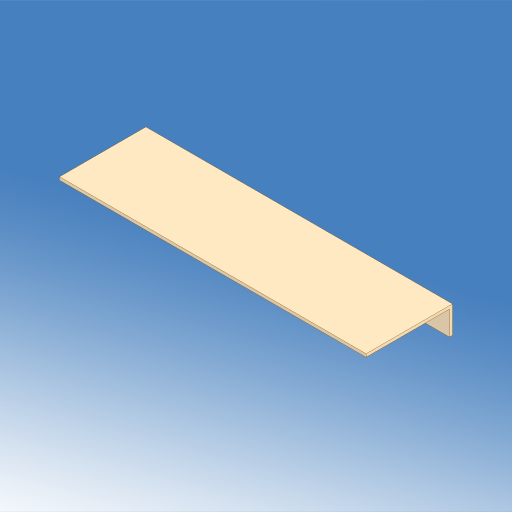
# Autodesk Inventor part: flat chain guide
Saved by Autodesk Inventor 2024 (Build 280153000, 153)
## iProperties
Created: 2023-03-01
Part Number: flat chain guide
Material: Polyethylene, High Density
Document SubType Name: Modeling
Designer: ralph
Density: 0.952 g/cm^3
Appearance: Smooth - Off-White
Author: ralph
Autodesk Inventor part; units mm, degrees
ref_plane "Work Plane1" through (-105.5469, -33.8995, 0) normal (0, 0, 1) x (1, 0, 0)
sketch "Sketch1" plane through (-105.5469, -33.8995, 0) normal (0, 0, 1) x (1, 0, 0)
  circle A0 centre (51.4164, 20.6909) radius 2.413 projected
  circle A1 centre (61.5426, -29.0897) radius 2.413 projected
  circle A2 centre (41.2902, 70.4714) radius 2.413 projected
  circle A3 centre (71.6688, -78.8702) radius 2.413 projected
  circle A4 centre (27.8827, -36.0288) radius 3.175 projected
  line L0 (21.5564, -145.7309) -> (-91.4082, 76.2381) projected
  line L1 (59.5069, 74.2446) -> (98.755, -118.7966) projected
  line L2 (15.2228, 144.056) -> (44.9436, 105.9012) projected
  line L3 (63.6348, -131.723) -> (58.903, -119.9375) projected
  line L4 (53.0129, -122.3028) -> (57.7447, -134.0883) projected
  arc A5 (3.7348, 135.3868) -> (-79.7406, 82.2913) centre (-35.4587, 104.8391) ccw
  line L5 (3.7348, 135.3868) -> (33.4679, 97.2384)
  arc A6 (45.3974, 71.3204) -> (33.4679, 97.2384) centre (-15.7425, 58.8835) ccw
  line L6 (45.3974, 71.3204) -> (84.6647, -121.7179)
  arc A7 (33.2723, -139.6562) -> (84.6647, -121.7179) centre (57.7489, -127.193) ccw
  arc A8 (2.9524, 134.777) -> (-78.8566, 82.7414) centre (-35.4587, 104.8391) ccw
  line L7 (2.9524, 134.777) -> (32.6855, 96.6286)
  arc A9 (44.4253, 71.1227) -> (32.6855, 96.6286) centre (-15.7425, 58.8835) ccw
  line L8 (44.4253, 71.1227) -> (83.6926, -121.9156)
  arc A10 (34.1563, -139.2061) -> (83.6926, -121.9156) centre (57.7489, -127.193) ccw
  line L9 (34.1563, -139.2061) -> (-78.8566, 82.7414)
  arc A11 (-4.5602, 128.9216) -> (-70.3686, 87.0634) centre (-35.4587, 104.8391) ccw
  line L10 (-4.5602, 128.9216) -> (25.1729, 90.7732)
  arc A12 (35.0915, 69.224) -> (25.1729, 90.7732) centre (-15.7425, 58.8835) ccw
  line L11 (35.0915, 69.224) -> (74.3588, -123.8143)
  arc A13 (42.6443, -134.8841) -> (74.3588, -123.8143) centre (57.7489, -127.193) ccw
  line L12 (42.6443, -134.8841) -> (-70.3686, 87.0634)
  arc A14 (5.4566, 136.7288) -> (-81.686, 81.3007) centre (-35.4587, 104.8391) ccw
  line L13 (5.4566, 136.7288) -> (35.1897, 98.5804)
  arc A15 (47.5366, 71.7556) -> (35.1897, 98.5804) centre (-15.7425, 58.8835) ccw
  line L14 (47.5366, 71.7556) -> (86.8039, -121.2827)
  arc A16 (31.327, -140.6467) -> (86.8039, -121.2827) centre (57.7489, -127.193) ccw
  line L15 (31.327, -140.6467) -> (-81.686, 81.3007)
  circle A17 centre (57.7489, -127.193) radius 44.45
  circle A18 centre (-35.4587, 104.8391) radius 69.85
  circle A19 centre (-47.8242, 28.7936) radius 2.413 projected
  circle A20 centre (-15.5534, -34.5834) radius 2.413 projected
  circle A21 centre (16.7174, -97.9605) radius 2.413 projected
  line L16 (-33.1344, 24.0942) -> (34.7456, 18.5458) projected
  line L17 (36.5081, 12.9323) -> (-6.2049, -22.3208) projected
  line L18 (-20.7511, -20.2117) -> (-39.1333, 15.9083) projected
  line L19 (38.3036, 25.8999) -> (-20.4951, 30.706) projected
  line L20 (-21.5821, 36.7465) -> (30.7819, 61.2351) projected
  line L21 (44.0707, 55.5202) -> (48.097, 35.7165) projected
  line L22 (-53.0081, 43.1715) -> (-61.3301, 59.5239) projected
  line L23 (17.8998, 109.9146) -> (30.1007, 94.2514) projected
  line L24 (27.5547, 68.1378) -> (-5.8444, 52.5185) projected
  line L25 (27.1825, -114.3985) -> (25.3807, -110.8581) projected
  line L26 (32.1964, -96.6363) -> (38.137, -94.5724) projected
  line L27 (74.4344, -93.8236) -> (75.2107, -97.6416) projected
  line L28 (50.495, -96.7953) -> (49.4394, -94.1661) projected
  line L29 (51.3425, -89.9843) -> (60.23, -86.8964) projected
  line L30 (-10.1341, 54.212) -> (-12.6231, 60.4113) projected
  line L31 (-19.6913, 57.573) -> (-16.9128, 50.6526) projected
  line L32 (-18.5132, 46.5938) -> (-35.734, 38.5403) projected
  line L33 (42.124, -96.3889) -> (43.4268, -99.6336) projected
  arc A22 (40.3328, 7.2327) -> (41.7343, 8.6241) centre (33.4597, 15.5569) ccw projected
  arc A23 (45.6191, 9.409) -> (41.7343, 8.6241) centre (44.1679, 6.585) ccw projected
  arc A24 (45.6191, 9.409) -> (50.3997, 8.0475) centre (51.4164, 20.6909) ccw projected
  arc A25 (53.2564, 5.5162) -> (50.3997, 8.0475) centre (50.1452, 4.8827) ccw projected
  line L34 (53.2564, 5.5162) -> (57.2026, -13.8642) projected
  arc A26 (55.534, -17.3261) -> (57.2026, -13.8642) centre (54.0915, -14.4977) ccw projected
  arc A27 (55.534, -17.3261) -> (49.5198, -23.895) centre (61.311, -28.6529) ccw projected
  arc A28 (46.8024, -25.8738) -> (49.5198, -23.895) centre (46.5755, -22.7069) ccw projected
  line L35 (46.8024, -25.8738) -> (37.6772, -26.5277) projected
  arc A29 (35.5367, -25.8944) -> (37.6772, -26.5277) centre (37.4502, -23.3608) ccw projected
  arc A30 (35.5367, -25.8944) -> (18.8618, -27.0893) centre (27.8827, -36.0288) ccw projected
  arc A31 (16.8336, -28.0213) -> (18.8618, -27.0893) centre (16.6066, -24.8545) ccw projected
  line L36 (16.8336, -28.0213) -> (0.7655, -29.1728) projected
  arc A32 (-0.3587, -26.3652) -> (0.7655, -29.1728) centre (0.652, -27.5893) ccw projected
  line L37 (-0.3587, -26.3652) -> (40.3328, 7.2327) projected
  arc A33 (12.0706, -61.7398) -> (8.1483, -51.9706) centre (20.8352, -52.5488) ccw projected
  line L38 (25.9855, -70.6908) -> (17.4507, -83.8024) projected
  line L39 (11.5059, -83.5949) -> (-6.8763, -47.4749) projected
  line L40 (-0.2859, -37.1185) -> (-0.1921, -37.1119) projected
  line L41 (74.8789, -123.628) -> (78.6564, -122.8604) projected
  line L42 (0.38, 132.4063) -> (2.0588, 130.251) projected
  line L43 (38.7029, -137.0353) -> (37.8849, -135.428) projected
  line L44 (38.579, -133.2932) -> (44.3373, -130.3617) projected
  line L45 (12.0706, -61.7398) -> (13.7631, -65.9552) projected
  line L46 (17.8911, -67.7189) -> (22.1428, -66.0115) projected
  line L47 (2.9792, -39.0961) -> (8.1483, -51.9706) projected
  ellipse E0 centre (-34.8429, 105.035) end of major axis (-54.1736, 165.5211) minor radius 63.4728 (15.2228, 144.056) -> (-91.4082, 76.2381) ccw projected
  ellipse E1 centre (58.3238, -127.0129) end of major axis (45.7589, -87.6969) minor radius 41.2573 (21.5564, -145.7309) -> (98.755, -118.7966) ccw projected
  ellipse E2 centre (-15.1352, 59.076) end of major axis (-38.3321, 131.6593) minor radius 76.1674 (59.5069, 74.2446) -> (44.9436, 105.9012) ccw projected
  ellipse E3 centre (-34.8429, 105.035) end of major axis (-38.9507, 117.8883) minor radius 13.488 projected
  ellipse E4 centre (60.6898, -132.9057) end of major axis (59.7232, -129.8814) minor radius 3.1736 (57.7447, -134.0883) -> (63.6348, -131.723) ccw projected
  ellipse E5 centre (55.9579, -121.1202) end of major axis (54.9914, -118.0958) minor radius 3.1736 (58.903, -119.9375) -> (53.0129, -122.3028) ccw projected
  ellipse E6 centre (-47.0283, 29.0524) end of major axis (-50.8944, 41.1496) minor radius 12.6946 (-38.4497, 19.689) -> (-36.1193, 22.5544) ccw projected
  ellipse E7 centre (-33.3921, 20.9299) end of major axis (-34.3586, 23.9542) minor radius 3.1736 (-33.1344, 24.0942) -> (-36.1193, 22.5544) ccw projected
  ellipse E8 centre (34.4879, 15.3814) end of major axis (33.5214, 18.4057) minor radius 3.1736 (36.5081, 12.9323) -> (34.7456, 18.5458) ccw projected
  ellipse E9 centre (-8.2251, -19.8717) end of major axis (-7.2586, -22.896) minor radius 3.1736 (-9.5343, -22.7635) -> (-6.2049, -22.3208) ccw projected
  ellipse E10 centre (-14.7713, -34.3308) end of major axis (-18.6374, -22.2336) minor radius 12.6946 (-9.5343, -22.7635) -> (-17.2925, -21.8836) ccw projected
  ellipse E11 centre (-17.9228, -18.7718) end of major axis (-16.9563, -21.7962) minor radius 3.1736 (-20.7511, -20.2117) -> (-17.2925, -21.8836) ccw projected
  ellipse E12 centre (-36.305, 17.3481) end of major axis (-35.3385, 14.3238) minor radius 3.1736 (-38.4497, 19.689) -> (-39.1333, 15.9083) ccw projected
  ellipse E13 centre (38.5613, 29.0642) end of major axis (39.5278, 26.0399) minor radius 3.1736 (38.3036, 25.8999) -> (41.2885, 27.4397) ccw projected
  ellipse E14 centre (-20.2374, 33.8704) end of major axis (-19.2708, 30.8461) minor radius 3.1736 (-21.5821, 36.7465) -> (-20.4951, 30.706) ccw projected
  ellipse E15 centre (32.1266, 58.3589) end of major axis (31.1601, 61.3832) minor radius 3.1736 (34.1165, 60.8317) -> (30.7819, 61.2351) ccw projected
  ellipse E16 centre (42.0762, 70.723) end of major axis (38.2101, 82.8202) minor radius 12.6946 (34.1165, 60.8317) -> (41.1837, 58.0551) ccw projected
  ellipse E17 centre (40.9606, 54.8882) end of major axis (39.994, 57.9125) minor radius 3.1736 (44.0707, 55.5202) -> (41.1837, 58.0551) ccw projected
  ellipse E18 centre (44.9869, 35.0845) end of major axis (44.0204, 38.1088) minor radius 3.1736 (46.4291, 32.2559) -> (48.097, 35.7165) ccw projected
  ellipse E19 centre (-37.0786, 41.4165) end of major axis (-36.1121, 38.3922) minor radius 3.1736 (-39.0686, 38.9437) -> (-35.734, 38.5403) ccw projected
  ellipse E20 centre (-47.0283, 29.0524) end of major axis (-50.8944, 41.1496) minor radius 12.6946 (-39.0686, 38.9437) -> (-49.5495, 41.4996) ccw projected
  ellipse E21 centre (-50.1798, 44.6113) end of major axis (-49.2133, 41.587) minor radius 3.1736 (-53.0081, 43.1715) -> (-49.5495, 41.4996) ccw projected
  ellipse E22 centre (-58.5019, 60.9637) end of major axis (-57.5353, 57.9394) minor radius 3.1736 (-56.9933, 63.7566) -> (-61.3301, 59.5239) ccw projected
  ellipse E23 centre (-34.666, 105.0915) end of major axis (-48.9707, 149.8513) minor radius 46.9699 (-11.2596, 64.347) -> (12.228, 107.7818) ccw projected
  ellipse E24 centre (15.3966, 107.9636) end of major axis (14.43, 110.9879) minor radius 3.1736 (17.8998, 109.9146) -> (12.228, 107.7818) ccw projected
  ellipse E25 centre (-14.9584, 59.1325) end of major axis (2.4393, 4.6949) minor radius 57.1256 (35.8618, 85.223) -> (30.1007, 94.2514) ccw projected
  ellipse E26 centre (33.0385, 83.7735) end of major axis (32.0719, 86.7978) minor radius 3.1736 (34.846, 81.1634) -> (35.8618, 85.223) ccw projected
  ellipse E27 centre (42.0762, 70.723) end of major axis (38.2101, 82.8202) minor radius 12.6946 (34.846, 81.1634) -> (29.3832, 70.9558) ccw projected
  ellipse E28 centre (26.21, 71.014) end of major axis (25.2435, 74.0383) minor radius 3.1736 (27.5547, 68.1378) -> (29.3832, 70.9558) ccw projected
  ellipse E29 centre (58.5007, -126.9564) end of major axis (49.8019, -99.7376) minor radius 28.5628 (70.7406, -101.1419) -> (53.9461, -98.747) ccw projected
  ellipse E30 centre (30.0108, -112.9586) end of major axis (30.9773, -115.9829) minor radius 3.1736 (27.1825, -114.3985) -> (32.8598, -114.3584) ccw projected
  ellipse E31 centre (28.209, -109.4182) end of major axis (29.1755, -112.4425) minor radius 3.1736 (26.0643, -107.0774) -> (25.3807, -110.8581) ccw projected
  ellipse E32 centre (17.4857, -97.714) end of major axis (21.3519, -109.8112) minor radius 12.6946 (26.0643, -107.0774) -> (30.0878, -99.2512) ccw projected
  ellipse E33 centre (33.2384, -99.6355) end of major axis (34.2049, -102.6598) minor radius 3.1736 (32.1964, -96.6363) -> (30.0878, -99.2512) ccw projected
  ellipse E34 centre (61.272, -89.8956) end of major axis (60.3054, -86.8713) minor radius 3.1736 (63.5056, -87.6406) -> (60.23, -86.8964) ccw projected
  ellipse E35 centre (72.44, -78.6208) end of major axis (68.5739, -66.5236) minor radius 12.6946 (63.5056, -87.6406) -> (71.5475, -91.2887) ccw projected
  ellipse E36 centre (71.3244, -94.4556) end of major axis (70.3578, -91.4313) minor radius 3.1736 (74.4344, -93.8236) -> (71.5475, -91.2887) ccw projected
  ellipse E37 centre (72.1006, -98.2736) end of major axis (73.0671, -101.2979) minor radius 3.1736 (70.7406, -101.1419) -> (75.2107, -97.6416) ccw projected
  ellipse E38 centre (58.5007, -126.9564) end of major axis (49.8019, -99.7376) minor radius 28.5628 (42.2836, -103.4303) -> (32.8598, -114.3584) ccw projected
  ellipse E39 centre (-34.666, 105.0915) end of major axis (-48.9707, 149.8513) minor radius 46.9699 (-56.9933, 63.7566) -> (-23.3977, 59.4727) ccw projected
  ellipse E40 centre (53.44, -95.6126) end of major axis (54.4066, -98.6369) minor radius 3.1736 (50.495, -96.7953) -> (53.9461, -98.747) ccw projected
  ellipse E41 centre (52.3844, -92.9835) end of major axis (53.351, -96.0078) minor radius 3.1736 (51.3425, -89.9843) -> (49.4394, -94.1661) ccw projected
  ellipse E42 centre (-7.1891, 55.3946) end of major axis (-6.2225, 52.3703) minor radius 3.1736 (-10.1341, 54.212) -> (-5.8444, 52.5185) ccw projected
  ellipse E43 centre (-9.6781, 61.594) end of major axis (-8.7115, 58.5697) minor radius 3.1736 (-11.2596, 64.347) -> (-12.6231, 60.4113) ccw projected
  ellipse E44 centre (-19.8578, 49.4699) end of major axis (-20.8244, 52.4943) minor radius 3.1736 (-18.5132, 46.5938) -> (-16.9128, 50.6526) ccw projected
  ellipse E45 centre (-22.6364, 56.3903) end of major axis (-23.6029, 59.4146) minor radius 3.1736 (-19.6913, 57.573) -> (-23.3977, 59.4727) ccw projected
  ellipse E46 centre (39.179, -97.5715) end of major axis (38.2124, -94.5472) minor radius 3.1736 (42.124, -96.3889) -> (38.137, -94.5724) ccw projected
  ellipse E47 centre (40.4817, -100.8163) end of major axis (39.5152, -97.792) minor radius 3.1736 (42.2836, -103.4303) -> (43.4268, -99.6336) ccw projected
  ellipse E48 centre (14.791, -82.0695) end of major axis (15.7575, -85.0938) minor radius 3.1736 (15.3299, -85.1984) -> (17.4507, -83.8024) ccw projected
  ellipse E49 centre (17.4857, -97.714) end of major axis (13.6196, -85.6168) minor radius 12.6946 (15.3299, -85.1984) -> (14.9645, -85.2668) ccw projected
  ellipse E50 centre (14.3342, -82.155) end of major axis (15.3007, -85.1793) minor radius 3.1736 (11.5059, -83.5949) -> (14.9645, -85.2668) ccw projected
  ellipse E51 centre (-4.048, -46.035) end of major axis (-3.0815, -49.0593) minor radius 3.1736 (-6.1927, -43.6942) -> (-6.8763, -47.4749) ccw projected
  ellipse E52 centre (-14.7713, -34.3308) end of major axis (-10.9051, -46.428) minor radius 12.6946 (-6.1927, -43.6942) -> (-3.002, -39.0945) ccw projected
  ellipse E53 centre (-0.0597, -40.2854) end of major axis (-1.0262, -37.2611) minor radius 3.1736 (-0.2859, -37.1185) -> (-3.002, -39.0945) ccw projected
  ellipse E54 centre (-75.9068, 106.3278) end of major axis (-76.8733, 109.3521) minor radius 3.1736 (-73.3969, 108.2703) -> (-79.0792, 106.4229) ccw projected
  ellipse E55 centre (-58.3372, 119.9252) end of major axis (-64.1365, 138.071) minor radius 19.0419 (-73.3969, 108.2703) -> (-70.1692, 105.0022) ccw projected
  ellipse E56 centre (-72.1411, 102.5151) end of major axis (-73.1077, 105.5394) minor radius 3.1736 (-69.8464, 100.3213) -> (-70.1692, 105.0022) ccw projected
  ellipse E57 centre (-56.078, 87.1583) end of major axis (-61.8772, 105.3042) minor radius 19.0419 (-69.8464, 100.3213) -> (-72.5951, 96.6423) ccw projected
  ellipse E58 centre (-75.348, 98.223) end of major axis (-74.3814, 95.1987) minor radius 3.1736 (-78.4773, 97.6947) -> (-72.5951, 96.6423) ccw projected
  ellipse E59 centre (-34.666, 105.0915) end of major axis (-21.1345, 62.7512) minor radius 44.431 (-79.0792, 106.4229) -> (-78.4773, 97.6947) ccw projected
  ellipse E60 centre (-46.2445, 144.7092) end of major axis (-47.211, 147.7336) minor radius 3.1736 (-43.6215, 142.9211) -> (-47.1351, 147.7568) ccw projected
  ellipse E61 centre (-27.8837, 132.1924) end of major axis (-33.6829, 150.3383) minor radius 19.0419 (-43.6215, 142.9211) -> (-45.7303, 138.8412) ccw projected
  ellipse E62 centre (-48.7048, 139.9494) end of major axis (-47.7382, 136.925) minor radius 3.1736 (-50.0809, 137.0888) -> (-45.7303, 138.8412) ccw projected
  ellipse E63 centre (-58.3372, 119.9252) end of major axis (-64.1365, 138.071) minor radius 19.0419 (-50.0809, 137.0888) -> (-54.4286, 138.5679) ccw projected
  ellipse E64 centre (-53.7771, 141.675) end of major axis (-52.8106, 138.6507) minor radius 3.1736 (-55.2472, 144.4891) -> (-54.4286, 138.5679) ccw projected
  ellipse E65 centre (-34.666, 105.0915) end of major axis (-21.1345, 62.7512) minor radius 44.431 (-47.1351, 147.7568) -> (-55.2472, 144.4891) ccw projected
  ellipse E66 centre (78.9727, -124.4161) end of major axis (78.4894, -122.9039) minor radius 1.5868 (80.5474, -124.2206) -> (78.6564, -122.8604) ccw projected
  ellipse E67 centre (58.5007, -126.9564) end of major axis (51.735, -105.7862) minor radius 22.2155 (79.7691, -133.3844) -> (80.5474, -124.2206) ccw projected
  ellipse E68 centre (76.7308, -132.4661) end of major axis (77.6973, -135.4904) minor radius 3.1736 (73.5579, -132.5427) -> (79.7691, -133.3844) ccw projected
  ellipse E69 centre (60.8666, -132.8492) end of major axis (64.7328, -144.9464) minor radius 12.6946 (73.5579, -132.5427) -> (72.5825, -127.9613) ccw projected
  ellipse E70 centre (75.5115, -126.7394) end of major axis (74.545, -123.7151) minor radius 3.1736 (74.8789, -123.628) -> (72.5825, -127.9613) ccw projected
  ellipse E71 centre (-0.4445, 128.2999) end of major axis (0.522, 125.2756) minor radius 3.1736 (-1.3529, 125.2581) -> (2.0588, 130.251) ccw projected
  ellipse E72 centre (-6.8031, 107.0071) end of major axis (-12.6023, 125.153) minor radius 19.0419 (-1.3529, 125.2581) -> (-6.001, 126.0393) ccw projected
  ellipse E73 centre (-5.8673, 129.2113) end of major axis (-4.9008, 126.187) minor radius 3.1736 (-9.0125, 129.6372) -> (-6.001, 126.0393) ccw projected
  ellipse E74 centre (-27.8837, 132.1924) end of major axis (-33.6829, 150.3383) minor radius 19.0419 (-9.0125, 129.6372) -> (-8.9508, 134.2302) ccw projected
  ellipse E75 centre (-5.7954, 134.5699) end of major axis (-6.7619, 137.5942) minor radius 3.1736 (-3.5745, 136.8374) -> (-8.9508, 134.2302) ccw projected
  ellipse E76 centre (-34.666, 105.0915) end of major axis (-21.1345, 62.7512) minor radius 44.431 (0.38, 132.4063) -> (-3.5745, 136.8374) ccw projected
  ellipse E77 centre (39.299, -134.708) end of major axis (39.7823, -136.2202) minor radius 1.5868 (38.579, -133.2932) -> (37.8849, -135.428) ccw projected
  ellipse E78 centre (45.0573, -131.7765) end of major axis (44.5741, -130.2644) minor radius 1.5868 (46.551, -131.2409) -> (44.3373, -130.3617) ccw projected
  ellipse E79 centre (58.5007, -126.9564) end of major axis (54.6346, -114.8592) minor radius 12.6946 (46.551, -131.2409) -> (48.2775, -134.4832) ccw projected
  ellipse E80 centre (60.8666, -132.8492) end of major axis (64.7328, -144.9464) minor radius 12.6946 (48.2775, -134.4832) -> (51.4877, -141.4055) ccw projected
  ellipse E81 centre (49.1429, -143.5446) end of major axis (48.1764, -140.5202) minor radius 3.1736 (47.5833, -146.3092) -> (51.4877, -141.4055) ccw projected
  ellipse E82 centre (58.5007, -126.9564) end of major axis (51.735, -105.7862) minor radius 22.2155 (38.7029, -137.0353) -> (47.5833, -146.3092) ccw projected
  ellipse E83 centre (52.1975, 20.9417) end of major axis (48.3314, 33.0389) minor radius 12.6946 (46.4291, 32.2559) -> (41.2885, 27.4397) ccw projected
  ellipse E84 centre (16.7081, -64.7725) end of major axis (17.6747, -67.7968) minor radius 3.1736 (13.7631, -65.9552) -> (17.8911, -67.7189) ccw projected
  ellipse E85 centre (23.3258, -68.9579) end of major axis (22.3593, -65.9336) minor radius 3.1736 (25.9855, -70.6908) -> (22.1428, -66.0115) ccw projected
  ellipse E86 centre (0.0342, -40.2787) end of major axis (-0.9324, -37.2544) minor radius 3.1736 (2.9792, -39.0961) -> (-0.1921, -37.1119) ccw projected
  ellipse E87 centre (45.8902, -59.8967) end of major axis (44.9237, -56.8724) minor radius 3.1736 (44.7072, -56.9504) -> (43.2305, -58.1638) ccw projected
  line L48 (44.7072, -56.9504) -> (46.8705, -56.0816) projected
  ellipse E88 centre (45.6876, -53.1353) end of major axis (44.721, -50.111) minor radius 3.1736 (46.8705, -56.0816) -> (48.6792, -52.0758) ccw projected
  ellipse E89 centre (51.6707, -51.0164) end of major axis (50.7042, -47.9921) minor radius 3.1736 (49.011, -49.2835) -> (48.6792, -52.0758) ccw projected
  line L49 (49.011, -49.2835) -> (53.8355, -41.872) projected
  line L50 (25.969, -84.6816) -> (43.2305, -58.1638) projected
  ellipse E90 centre (-17.6922, -49.6994) end of major axis (-15.8961, -55.3194) minor radius 5.8975 (-22.8057, -52.6378) -> (-14.6753, -44.6307) ccw projected
  ellipse E91 centre (-17.6417, -49.6706) end of major axis (-16.9644, -51.79) minor radius 2.224 projected
  ellipse E92 centre (56.4952, -43.6049) end of major axis (55.5287, -40.5806) minor radius 3.1736 (57.6599, -40.6518) -> (53.8355, -41.872) ccw projected
  ellipse E93 centre (62.3188, -28.8395) end of major axis (58.4526, -16.7423) minor radius 12.6946 (57.6599, -40.6518) -> (61.4262, -41.5074) ccw projected
  ellipse E94 centre (61.2031, -44.6744) end of major axis (60.2366, -41.6501) minor radius 3.1736 (64.3132, -44.0423) -> (61.4262, -41.5074) ccw projected
  line L51 (64.3132, -44.0423) -> (68.3396, -63.846) projected
  ellipse E95 centre (65.2295, -64.478) end of major axis (64.2629, -61.4537) minor radius 3.1736 (66.6716, -67.3066) -> (68.3396, -63.846) ccw projected
  ellipse E96 centre (72.44, -78.6208) end of major axis (68.5739, -66.5236) minor radius 12.6946 (66.6716, -67.3066) -> (59.8379, -77.0836) ccw projected
  ellipse E97 centre (56.6874, -76.6993) end of major axis (55.7209, -73.675) minor radius 3.1736 (57.7293, -79.6984) -> (59.8379, -77.0836) ccw projected
  line L52 (57.7293, -79.6984) -> (29.6957, -89.4384) projected
  ellipse E98 centre (28.6538, -86.4392) end of major axis (29.6203, -89.4635) minor radius 3.1736 (26.4202, -88.6942) -> (29.6957, -89.4384) ccw projected
  ellipse E99 centre (17.4857, -97.714) end of major axis (21.3519, -109.8112) minor radius 12.6946 (26.4202, -88.6942) -> (26.4002, -88.6744) ccw projected
  ellipse E100 centre (28.6288, -86.4145) end of major axis (27.6622, -83.3902) minor radius 3.1736 (25.969, -84.6816) -> (26.4002, -88.6744) ccw projected
  point P0 (105.5469, 33.8995)
  point P1 (-44.128, 35.5292)
  point P2 (-60.4612, 39.6172)
  point P3 (16.3005, -111.136)
  point P4 (23.999, -98.2664)
  point P5 (-35.4703, 104.8623)
  point P6 (57.7373, -127.1698)
  dimension "d0" = 12.7
  dimension "d1" = 9.525
  dimension "d2" = 88.9
  dimension "d3" = 139.7
  constraints: 24 point on circle, 22 end point, 14 centre point, 1 coincident, 120 other
  measures "d0" distance between parallel lines of L15 L12
  measures "d1" distance between parallel lines of L9 L12
  measures "d2" diameter of A17
  measures "d3" diameter of A18
ref_plane "Work Plane2" through (-41.9854, -105.2288, 43.0784) normal (0, 0, 1) x (1, 0, 0)
extrude "Extrusion1" add sketch "Sketch1" along normal up to surface (43.0784 mm away) contours L15 E90 L9 A17 | A18 L9 E90 L15 | L9 E90 A18 L12 E6 E12 L18 E11 E10 E52 E51 L39 E50 E49 E48 A17 | L9 E90 | E48 E49 E50 L39 E51 E52 L12 | L12 E10 E11 L18 E12 E6 | A19 | A20 | A21
sketch "Sketch2" plane through (-166.0081, 5.7177, 0) normal (-0.8911282, -0.4537516, 0) x (0, 0, 1)
  spline S0 degree 3 number of poles 454
  line L0 (43.0784, -169.1712) -> (43.0784, 0)
  line L1 (0, 0) -> (43.0784, 0)
  line L2 (0, 0) -> (0, -169.1712)
  line L3 (0, -169.1712) -> (43.0784, -169.1712)
  line L4 (13.1572, -174.2662) -> (29.9212, -174.2662)
  line L5 (13.1572, -174.2662) -> (13.1572, -19.5178)
  line L6 (13.1572, -19.5178) -> (29.9212, -19.5178)
  line L7 (29.9212, -19.5178) -> (29.9212, -174.2662)
  line L8 (13.1572, -19.5178) -> (13.1572, 0)
  line L9 (29.9212, -19.5178) -> (29.9212, 0)
  point P0 (0, -80.4217)
  point P1 (13.1572, -169.1712)
  point P2 (29.9212, -169.1712)
  constraints: 4 end point, 2 perpendicular, 2 point on line
extrude "Extrusion2" cut sketch "Sketch2" against normal blind 3.175 contours L3 L5 L6 L7 | L9 L6 L8 L1
fillet "Fillet1" radius 3.175 5 edges at (-89.2464, -145.0355, 6.5786) (-89.2464, -145.0355, 36.4998) (-81.5478, -132.1659, 21.5392) (-149.6749, 1.6297, 21.5392) (-166.0081, 5.7177, 6.5786)
sketch "Sketch3" plane through (-92.183, -139.2682, 43.0784) normal (0, 0, 1) x (0.8911282, 0.4537516, 0)
  line L0 (6.35, 5.08) -> (6.35, 156.499)
  arc A0 (5.2924, 157.4265) -> (11.3663, 152.5714) centre (51.875, 209.4754) ccw projected
  circle A1 centre (6.35, 5.08) radius 2.413
  arc A2 (0, 0) -> (4.94, -2.6392) centre (3.175, 0) ccw projected
  circle A3 centre (6.35, 76.2) radius 2.413
  circle A4 centre (6.35, 147.32) radius 2.413
  point P0 (145.3401, 82.2776)
  dimension "d9" = 4.826
  dimension "d10" = 5.08
  dimension "d13" = 71.12
  constraints: 3 centre point, 2 end point, 2 vertical, 1 coincident, 1 point on circle, 4 other
  measures "d9" diameter of A1
  measures "d10" vertical distance of A2.centre L0.start
  measures "d13" distance of A1.centre A3.centre
ref_plane "Work Plane3" through (-228.5882, -244.5835, 0) normal (0, 0, 1) x (1, 0, 0)
extrude "Extrusion3" cut sketch "Sketch3" against normal up to surface (43.0784 mm away)
thread "Thread1" size "10-24 UNC" class "2B" standard "ANSI Unified Screw Threads" full length
thread "Thread2" size "10-24 UNC" class "2B" standard "ANSI Unified Screw Threads" full length
thread "Thread3" size "10-24 UNC" class "2B" standard "ANSI Unified Screw Threads" full length
sketch "Sketch4" plane through (-148.9216, 0.1502, 43.0784) normal (0.8911282, 0.4537516, 0) x (0, 0, -1)
  line L0 (0, 0) -> (43.0784, 0) projected
  line L1 (0, 0) -> (0, -146.409) projected
  line L2 (43.0784, -146.409) -> (0, -146.409) projected
  line L3 (43.0784, -146.409) -> (43.0784, 0) projected
  line L4 (0, 2.5865) -> (0, 0) projected
  line L5 (0, 0) -> (43.0784, 0) projected
  line L6 (43.0784, 0) -> (43.0784, 2.5865) projected
  line L7 (43.0784, 2.5865) -> (0, 2.5865) projected
  line L8 (13.1572, 5.0759) -> (0, 5.0759) projected
  line L9 (0, 5.0759) -> (0, 7.4417) projected
  line L10 (0, 7.4417) -> (43.0784, 7.4417) projected
  line L11 (43.0784, 7.4417) -> (43.0784, 5.0759) projected
  line L12 (43.0784, 5.0759) -> (29.9212, 5.0759) projected
  line L13 (29.9212, 5.0759) -> (29.9212, 8.2509) projected
  line L14 (29.9212, 8.2509) -> (13.1572, 8.2509) projected
  line L15 (13.1572, 8.2509) -> (13.1572, 5.0759) projected
  line L16 (13.1572, 5.0759) -> (0, 5.0759) projected
  line L17 (0, 7.4417) -> (43.0784, 7.4417) projected
  line L18 (0, 7.4417) -> (0, 2.5865) projected
  line L19 (43.0784, 2.5865) -> (0, 2.5865) projected
  line L20 (43.0784, 2.5865) -> (43.0784, 7.4417) projected
  line L21 (0, -152.624) -> (0, -149.9848) projected
  line L22 (0, -149.9848) -> (13.1572, -149.9848) projected
  line L23 (13.1572, -149.9848) -> (13.1572, -153.1598) projected
  line L24 (13.1572, -153.1598) -> (29.9212, -153.1598) projected
  line L25 (29.9212, -153.1598) -> (29.9212, -149.9848) projected
  line L26 (43.0784, -149.9848) -> (29.9212, -149.9848) projected
  line L27 (43.0784, -149.9848) -> (43.0784, -152.624) projected
  line L28 (43.0784, -152.624) -> (0, -152.624) projected
  line L29 (0, -149.2865) -> (43.0784, -149.2865) projected
  line L30 (0, -149.2865) -> (0, -152.624) projected
  line L31 (43.0784, -152.624) -> (0, -152.624) projected
  line L32 (43.0784, -152.624) -> (43.0784, -149.2865) projected
  line L33 (0, -146.409) -> (0, -149.2865) projected
  line L34 (0, -149.2865) -> (43.0784, -149.2865) projected
  line L35 (43.0784, -149.2865) -> (43.0784, -146.409) projected
  line L36 (43.0784, -146.409) -> (0, -146.409) projected
  line L37 (43.0784, -153.1598) -> (0, -153.1598) projected
  line L38 (0, -152.624) -> (0, -149.9848) projected
  line L39 (0, -149.9848) -> (13.1572, -149.9848) projected
  line L40 (13.1572, -149.9848) -> (13.1572, -153.1598) projected
  line L41 (13.1572, -153.1598) -> (29.9212, -153.1598) projected
  line L42 (29.9212, -153.1598) -> (29.9212, -149.9848) projected
  line L43 (43.0784, -149.9848) -> (29.9212, -149.9848) projected
  line L44 (43.0784, -149.9848) -> (43.0784, -152.624) projected
  line L45 (43.0784, -152.624) -> (0, -152.624) projected
  line L46 (0, -153.1598) -> (43.0784, -153.1598)
  line L47 (43.0784, -153.1598) -> (43.0784, 7.4417)
  line L48 (43.0784, 7.4417) -> (0, 7.4417)
  line L49 (0, 7.4417) -> (0, -153.1598)
  point P0 (43.0784, -67.7072)
  constraints: 8 end point, 2 parallel, 1 horizontal, 1 perpendicular
sketch "Sketch5" plane through (-92.183, -139.2682, 43.0784) normal (0, 0, 1) x (0.8911282, 0.4537516, 0)
  line L0 (12.7, 149.9848) -> (12.7, 3.5759) projected
  line L1 (3.175, 158.2357) -> (3.175, -3.175) projected
  circle A0 centre (6.35, 147.32) radius 2.413 projected
  circle A1 centre (6.35, 5.08) radius 2.413 projected
  circle A2 centre (6.35, 76.2) radius 2.413 projected
  arc A3 (5.2924, 157.4265) -> (0, 155.0607) centre (3.175, 155.0607) ccw projected
  line L2 (0, 0) -> (0, 155.0607) projected
  arc A4 (0, 0) -> (4.94, -2.6392) centre (3.175, 0) ccw projected
  arc A5 (10.8667, 0.6983) -> (4.94, -2.6392) centre (29.65, -39.5881) ccw projected
  arc A6 (10.8667, 0.6983) -> (12.7, 3.5759) centre (9.525, 3.5759) ccw projected
  line L3 (12.7, 149.9848) -> (12.7, 3.5759) projected
  arc A7 (12.7, 149.9848) -> (11.3663, 152.5714) centre (9.525, 149.9848) ccw projected
  arc A8 (5.2924, 157.4265) -> (11.3663, 152.5714) centre (51.875, 209.4754) ccw projected
  line L4 (0, -3.175) -> (12.7, -3.175)
  line L5 (12.7, -3.175) -> (12.7, 158.2357)
  line L6 (12.7, 158.2357) -> (0, 158.2357)
  line L7 (0, 158.2357) -> (0, -3.175)
  arc A9 (0, 0) -> (4.94, -2.6392) centre (3.175, 0) ccw projected
  arc A10 (5.2924, 157.4265) -> (0, 155.0607) centre (3.175, 155.0607) ccw projected
  line L8 (0, -3.175) -> (-1.5875, -3.175)
  line L9 (-1.5875, -3.175) -> (-1.5875, 158.2357)
  line L10 (-1.5875, 158.2357) -> (0, 158.2357)
  line L11 (0, 158.2357) -> (0, -3.175)
  point P0 (145.3401, 82.2776)
  point P1 (0, 0)
  point P2 (0, 158.2357)
  dimension "d28" = 1.5875
  constraints: 16 end point, 4 parallel, 2 collinear, 2 horizontal, 2 perpendicular, 2 tangent
  measures "d28" distance between parallel lines of L2 L9
extrude "Extrusion4" add sketch "Sketch5" along normal blind 1.5875 contours L0 A6 A5 A4 L1 A3 A8 A7 | A7 A8 A3 L6 L5 | L5 L4 A4 A5 A6 | L1 A4 L2 A3 | A3 L7 L6 | L4 L7 A4
extrude "Extrusion5" add sketch "Sketch5" along normal blind 45.4596 contours L2 L7 L8 L9 L10
extrude "Extrusion6" cut sketch "Sketch5" against normal blind 43.0784 contours L0 A6 A5 A4 L1 A3 A8 A7 | A7 A8 A3 L6 L5 | L5 L4 A4 A5 A6 | L1 A4 L2 A3 | A3 L7 L6 | L4 L7 A4 | A0 | A1 | A2
body "Solid1"
